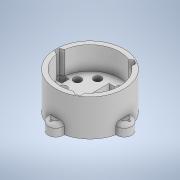
# Autodesk Inventor part: Enganche_H
Saved by Autodesk Inventor 2021 (Build 250183000, 183)
## iProperties
Created: 2021-10-28
Part Number: Enganche_H
Material: Genérico
Document SubType Name: Modeling
Designer: Joaquín
Density: 1 g/cm^3
Appearance: Valor por defecto
Author: Joaquín
Autodesk Inventor part; units mm, degrees
ref_plane "YZ Plane" through (0, 0, 0) normal (1, 0, 0) x (0, 1, 0)
ref_plane "XZ Plane" through (0, 0, 0) normal (0, 1, 0) x (-1, 0, 0)
ref_plane "XY Plane" through (0, 0, 0) normal (0, 0, 1) x (1, 0, 0)
sketch "Boceto3" plane through (0, 0, 0) normal (0, 1, 0) x (-1, 0, 0)
  line L0 (-22.9127, 29.686) -> (-23.0801, 29.976)
  line L1 (-23.0801, 29.976) -> (-22.6604, 29.249)
  line L2 (-19.0849, 38.0561) -> (-23.4151, 35.5561)
  line L3 (-23.0801, 29.976) -> (-23.4151, 35.5561)
  line L4 (-23.4151, 35.5561) -> (-19.0849, 38.0561)
  line L5 (-19.0849, 38.0561) -> (-14.4199, 34.976)
  line L6 (-14.4199, 34.976) -> (-14.0002, 34.249)
  line L7 (-22.6604, -29.249) -> (-23.0801, -29.976)
  line L8 (-22.6604, -29.249) -> (-23.0801, -29.976)
  line L9 (-23.0801, -29.976) -> (-23.4151, -35.5561)
  line L10 (-23.0801, -29.976) -> (-23.4151, -35.5561)
  line L11 (-23.4151, -35.5561) -> (-19.0849, -38.0561)
  line L12 (-23.4151, -35.5561) -> (-19.0849, -38.0561)
  line L13 (-19.0849, -38.0561) -> (-14.4199, -34.976)
  line L14 (-14.4199, -34.976) -> (-14.0002, -34.249)
  line L15 (-14.4199, -34.976) -> (-14.0002, -34.249)
  line L16 (36.6606, -5) -> (37.5, -5)
  line L17 (36.6606, -5) -> (37.5, -5)
  line L18 (37.5, -5) -> (42.5, -2.5)
  line L19 (37.5, -5) -> (42.5, -2.5)
  line L20 (42.5, 2.5) -> (37.5, 5)
  line L21 (42.5, -2.5) -> (42.5, 2.5)
  line L22 (42.5, 2.5) -> (37.5, 5)
  line L23 (37.5, 5) -> (36.6606, 5)
  line L24 (37.5, 5) -> (36.6606, 5)
  arc A0 (36.6606, 5) -> (-14.0002, 34.249) centre (0, 0) ccw
  arc A1 (-22.6604, 29.249) -> (-22.6604, -29.249) centre (0, 0) ccw
  arc A2 (-14.0002, -34.249) -> (36.6606, -5) centre (0, 0) ccw
  circle A3 centre (0, 0) radius 45
  point P0 (5, 25)
  dimension "d7" = 90
  constraints: 50 end point, 8 collinear, 6 point on circle, 4 centre point, 2 perpendicular, 1 coincident, 1 horizontal, 1 parallel
  measures "d7" diameter of A3
extrude "Extrusión2" add sketch "Boceto3" along normal blind 30
sketch "Boceto4" plane through (0, 0, 0) normal (0, -1, 0) x (1, 0, 0)
  circle A0 centre (0, 0) radius 45
  line L0 (-42.5, -2.5) -> (-37.5, -5) projected
  line L1 (-36.6606, -5) -> (-37.5, -5)
  line L2 (-37.5, -5) -> (-42.5, -2.5)
  line L3 (-42.5, 2.5) -> (-42.5, -2.5) projected
  line L4 (-42.5, -2.5) -> (-42.5, 2.5)
  line L5 (-37.5, 5) -> (-42.5, 2.5) projected
  line L6 (-42.5, 2.5) -> (-37.5, 5)
  line L7 (-37.5, 5) -> (-36.6606, 5)
  line L8 (14.4199, 34.976) -> (14.0002, 34.249) projected
  line L9 (14.0002, 34.249) -> (14.4199, 34.976)
  line L10 (19.0849, 38.0561) -> (14.4199, 34.976) projected
  line L11 (14.4199, 34.976) -> (19.0849, 38.0561)
  line L12 (23.4151, 35.5561) -> (19.0849, 38.0561) projected
  line L13 (19.0849, 38.0561) -> (23.4151, 35.5561)
  line L14 (23.0801, 29.976) -> (23.4151, 35.5561) projected
  line L15 (23.4151, 35.5561) -> (23.0801, 29.976)
  line L16 (22.6604, 29.249) -> (23.0801, 29.976) projected
  line L17 (23.0801, 29.976) -> (22.6604, 29.249)
  line L18 (14.0002, -34.249) -> (14.4199, -34.976)
  line L19 (19.0849, -38.0561) -> (23.4151, -35.5561) projected
  line L20 (14.4199, -34.976) -> (19.0849, -38.0561)
  line L21 (19.0849, -38.0561) -> (23.4151, -35.5561)
  line L22 (23.4151, -35.5561) -> (23.0801, -29.976) projected
  line L23 (23.4151, -35.5561) -> (23.0801, -29.976)
  line L24 (23.0801, -29.976) -> (22.6604, -29.249)
  arc A1 (-36.6606, 5) -> (-36.6606, -5) centre (0, 0) ccw
  arc A2 (14.0002, -34.249) -> (22.6604, -29.249) centre (0, 0) ccw
  arc A3 (22.6604, 29.249) -> (14.0002, 34.249) centre (0, 0) ccw
  constraints: 30 end point, 12 equal length, 6 point on circle, 4 centre point, 2 coincident, 1 horizontal
extrude "Extrusión3" add sketch "Boceto4" along normal blind 10
sketch "Boceto5" plane through (0, -10, 0) normal (0, -1, 0) x (1, 0, 0)
  line L0 (0, 0) -> (0, 20)
  line L1 (0, 20) -> (20, 20)
  line L2 (20, 20) -> (20, -20)
  line L3 (20, -20) -> (0, -20)
  line L4 (0, -20) -> (0, 0)
  dimension "d12" = 20
  dimension "d13" = 20
  dimension "d14" = 40
  dimension "d15" = 20
  constraints: 10 end point, 2 perpendicular, 1 point on line, 1 vertical
  measures "d12" distance of L0.start L0.end
  measures "d13" distance of L0.end L1.end
  measures "d14" distance of L1.end L2.end
  measures "d15" distance of L2.end L3.end
extrude "Extrusión4" cut sketch "Boceto5" against normal blind 10
sketch "Boceto6" plane through (0, -10, 0) normal (0, -1, 0) x (1, 0, 0)
  line L0 (-36.6606, -5) -> (-32.1, -5)
  line L1 (-32.1, -5) -> (-32.1, 5)
  line L2 (-32.1, 5) -> (-36.6606, 5)
  arc A0 (-36.6606, 5) -> (-36.6606, -5) centre (0, 0) ccw
  line L3 (22.6604, -29.249) -> (20.3801, -25.2994)
  arc A1 (14.0002, -34.249) -> (22.6604, -29.249) centre (0, 0) ccw
  line L4 (20.3801, -25.2994) -> (11.7199, -30.2994)
  line L5 (11.7199, -30.2994) -> (14.0002, -34.249)
  line L6 (14.0002, 34.249) -> (11.7199, 30.2994)
  arc A2 (22.6604, 29.249) -> (14.0002, 34.249) centre (0, 0) ccw
  line L7 (11.7199, 30.2994) -> (20.3801, 25.2994)
  line L8 (20.3801, 25.2994) -> (22.6604, 29.249)
  dimension "d19" = 10
  dimension "d22" = 360
  constraints: 18 end point, 6 point on circle, 3 centre point, 2 perpendicular, 1 coincident, 28 other
  measures "d19" distance of L0.end L1.end
extrude "Extrusión5" cut sketch "Boceto6" against normal blind 10
sketch "Boceto7" plane through (0, -10, 0) normal (0, -1, 0) x (1, 0, 0)
  circle A0 centre (27.5, 0) radius 2.5
  circle A1 centre (21.0662, 17.6767) radius 2.5
  circle A2 centre (4.7753, 27.0822) radius 2.5
  circle A3 centre (-13.75, 23.8157) radius 2.5
  circle A4 centre (-25.8415, 9.4056) radius 2.5
  circle A5 centre (-25.8415, -9.4056) radius 2.5
  circle A6 centre (-13.75, -23.8157) radius 2.5
  circle A7 centre (4.7753, -27.0822) radius 2.5
  circle A8 centre (21.0662, -17.6767) radius 2.5
  circle A9 centre (-13.75, -23.8157) radius 5
  circle A10 centre (-25.8415, -9.4056) radius 5
  circle A11 centre (-25.8415, 9.4056) radius 5
  circle A12 centre (-13.75, 23.8157) radius 5
  point P0 (0, 0)
  dimension "d29" = 5
  dimension "d32" = 360
  dimension "d34" = 10
  dimension "d35" = 10
  constraints: 13 centre point, 4 coincident, 19 other
  measures "d29" diameter of A0
  measures "d34" diameter of A9
  measures "d35" diameter of A10
extrude "Extrusión6" cut sketch "Boceto7" against normal blind 10 contours A3 | A4 | A5 | A6 | A9 | A10 | A11 | A12
sketch "Boceto10" plane through (0, 0, 0) normal (0, 1, 0) x (1, 0, 0)
  line L0 (0, 20) -> (0, -20) projected
  arc A0 (14.8215, -21.6306) -> (5.3674, -21.5551) centre (10.1075, -19.9639) ccw
  arc A1 (7.6437, -28.3362) -> (12.4372, -28.3744) centre (10.0471, -27.5294) ccw
  line L1 (12.4658, -28.2937) -> (14.8215, -21.6306)
  line L2 (7.6356, -28.3119) -> (5.3674, -21.5551)
  line L3 (12.4372, -28.3744) -> (12.4658, -28.2937)
  line L4 (7.6437, -28.3362) -> (7.6356, -28.3119)
  line L5 (20, -20) -> (0, -20) projected
  line L6 (20, 20) -> (0, 20) projected
  arc A2 (5.1785, 21.6306) -> (14.6326, 21.5551) centre (9.8925, 19.9639) ccw
  arc A3 (12.3563, 28.3362) -> (7.5628, 28.3744) centre (9.9529, 27.5294) ccw
  line L7 (7.5342, 28.2937) -> (5.1785, 21.6306)
  line L8 (12.3644, 28.3119) -> (14.6326, 21.5551)
  line L9 (7.5628, 28.3744) -> (7.5342, 28.2937)
  line L10 (12.3563, 28.3362) -> (12.3644, 28.3119)
  point P0 (0, 0)
  point P1 (10, 0)
  point P2 (7.5628, 28.3744)
  dimension "d49" = 10
  dimension "d53" = 360
  constraints: 16 end point, 8 point on circle, 4 centre point, 4 point on line, 4 tangent, 31 other
  measures "d49" diameter of A0
extrude "Extrusión7" cut sketch "Boceto10" against normal blind 12
sketch "Boceto13" plane through (0, -10, 0) normal (0, -1, 0) x (1, 0, 0)
  arc A0 (31, 10) -> (10.1128, 30.9997) centre (10, 10) ccw
  arc A1 (10.1128, -30.9997) -> (31, -10) centre (10, -10) ccw
  arc A2 (-8.4662, 0) -> (-11, -10) centre (10, -10) ccw
  line L0 (0, -20) -> (0, 20) projected
  line L1 (0, 10) -> (0, -10)
  arc A3 (-11, 10) -> (-8.4662, 0) centre (10, 10) ccw
  arc A4 (-9.2351, 12.3895) -> (-11, 10) centre (-8.5, 10) ccw
  line L2 (-1.5423, 14.7562) -> (-9.2351, 12.3895)
  line L3 (0, 15) -> (0, 8.4662)
  arc A5 (0, 15) -> (-1.5423, 14.7562) centre (0, 10) ccw
  arc A6 (-11, -10) -> (-8.5, -12.5) centre (-8.5, -10) ccw
  line L4 (-1.5423, -14.7562) -> (-9.2351, -12.3895)
  line L5 (0, -10) -> (0, -15)
  arc A7 (-1.5423, -14.7562) -> (0, -15) centre (0, -10) ccw
  arc A8 (20, 5) -> (21.5423, 5.2438) centre (20, 10) ccw
  arc A9 (21.5423, -5.2438) -> (20, -5) centre (20, -10) ccw
  arc A10 (31, -10) -> (28.5, -7.5) centre (28.5, -10) ccw
  arc A11 (28.5, 7.5) -> (31, 10) centre (28.5, 10) ccw
  line L6 (21.5423, -5.2438) -> (29.2351, -7.6105)
  line L7 (20, 20) -> (15.1073, 20) projected
  line L8 (21.5423, 5.2438) -> (29.2351, 7.6105)
  line L9 (20, 5) -> (20, -5)
  line L10 (20, 20) -> (20, -20) projected
  circle A12 centre (0, 0) radius 45
  circle A13 centre (-13.75, 23.8157) radius 5 projected
  circle A14 centre (-13.75, 23.8157) radius 5
  circle A15 centre (-25.8415, 9.4056) radius 5 projected
  circle A16 centre (-25.8415, 9.4056) radius 5
  circle A17 centre (-25.8415, -9.4056) radius 5 projected
  circle A18 centre (-25.8415, -9.4056) radius 5
  circle A19 centre (-13.75, -23.8157) radius 5 projected
  circle A20 centre (-13.75, -23.8157) radius 5
  arc A21 (7.5628, -28.3744) -> (12.3563, -28.3362) centre (9.9529, -27.5294) ccw projected
  line L11 (0, 15) -> (0, 20)
  line L12 (0, 20) -> (5.1076, 20) projected
  line L13 (0, 20) -> (5.1076, 20)
  arc A22 (15.1073, 20) -> (14.8215, 21.6306) centre (10.1075, 19.9639) ccw projected
  arc A23 (16.1074, 20) -> (16.1034, 20.1849) centre (10.1075, 19.9639) ccw
  arc A24 (10.1128, 30.9997) -> (7.2499, 29.5844) centre (10.0471, 27.5294) ccw
  line L14 (6.5761, 27.5294) -> (4.1076, 20)
  line L15 (4.1076, 20) -> (7.2499, 29.5844)
  arc A25 (7.2499, -29.5844) -> (10.1128, -30.9997) centre (10.0471, -27.5294) ccw
  line L16 (4.1076, -20) -> (7.2499, -29.5844)
  line L17 (0, 15) -> (0, 20)
  line L18 (4.1076, 20) -> (0, 20)
  line L19 (0, -15) -> (0, -20)
  line L20 (0, -20) -> (4.1076, -20)
  line L21 (0, -20) -> (4.8927, -20) projected
  constraints: 34 end point, 30 point on circle, 20 centre point, 8 coincident, 8 point on line, 7 collinear, 4 tangent, 1 midpoint, 1 vertical
extrude "Extrusión8" add sketch "Boceto13" along normal blind 8
sketch "Boceto14" plane through (0, -18, 0) normal (0, -1, 0) x (1, 0, 0)
  circle A0 centre (0, 0) radius 45
  circle A1 centre (-13.75, -23.8157) radius 5 projected
  circle A2 centre (-13.75, -23.8157) radius 5
  circle A3 centre (-25.8415, -9.4056) radius 5 projected
  circle A4 centre (-25.8415, -9.4056) radius 5
  circle A5 centre (-25.8415, 9.4056) radius 5 projected
  circle A6 centre (-25.8415, 9.4056) radius 5
  circle A7 centre (-13.75, 23.8157) radius 5 projected
  circle A8 centre (-13.75, 23.8157) radius 5
  constraints: 5 centre point, 5 coincident
extrude "Extrusión9" add sketch "Boceto14" along normal blind 8
sketch "Boceto15" plane through (0, -26, 0) normal (0, -1, 0) x (1, 0, 0)
  line L0 (0, -35) -> (20, -35)
  line L1 (0, 35) -> (20, 35)
  line L2 (35, 0) -> (35, -10)
  line L3 (35, 0) -> (35, 10)
  line L4 (0, -35) -> (0, -30)
  line L5 (20, -35) -> (20, -30)
  line L6 (20, -30) -> (0, -30)
  line L7 (35, -10) -> (30, -10)
  line L8 (30, -10) -> (30, 10)
  line L9 (30, 10) -> (35, 10)
  line L10 (20, 35) -> (20, 30)
  line L11 (20, 30) -> (0, 30)
  line L12 (0, 30) -> (0, 35)
  dimension "d86" = 20
  dimension "d87" = 20
  dimension "d91" = 5
  dimension "d92" = 5
  dimension "d93" = 5
  dimension "d94" = 5
  constraints: 26 end point, 5 vertical, 4 perpendicular, 3 horizontal
  measures "d86" distance of L0.start L0.end
  measures "d87" distance of L1.start L1.end
  measures "d91" distance of L0.start L4.end
  measures "d92" distance of L0.end L5.end
  measures "d93" distance of L2.end L7.end
  measures "d94" distance of L1.end L10.end
extrude "Extrusión10" add sketch "Boceto15" along normal blind 20
sketch "Boceto17" plane through (0, -26, 35) normal (0, 0, 1) x (1, 0, 0)
  circle A0 centre (5, -15) radius 1.5
  circle A1 centre (15, -15) radius 1.5
  circle A2 centre (10, -5) radius 1.5
  point P0 (0, 26)
  point P1 (0, -20)
  dimension "d118" = 3
  constraints: 3 centre point
  measures "d118" diameter of A2
extrude "Extrusión11" cut sketch "Boceto17" against normal blind 100
sketch "Boceto19" plane through (35, -26, 10) normal (1, 0, 0) x (0, 0, -1)
  circle A0 centre (5, -15) radius 1.5
  circle A1 centre (15, -15) radius 1.5
  circle A2 centre (10, -5) radius 1.5
  point P0 (10, 26)
  point P1 (0, -20)
  dimension "d114" = 3
  dimension "d115" = 3
  dimension "d116" = 3
  constraints: 3 centre point
  measures "d114" diameter of A0
  measures "d115" diameter of A1
  measures "d116" diameter of A2
extrude "Extrusión12" cut sketch "Boceto19" against normal blind 100
fillet "Empalme1" radius 2 3 edges at (-18.5, 30, 32.0429) (37, 30, 0) (-18.5, 30, -32.0429)
sketch "Boceto22" plane through (0, -46, 0) normal (0, -1, 0) x (1, 0, 0)
  circle A0 centre (80.4507, 56.8705) radius 177.5507
  point P0 (0, 0)
  constraints: 1 centre point
extrude "Extrusión13" cut sketch "Boceto22" against normal blind 28
sketch "Boceto23" plane through (0, -18, 0) normal (0, -1, 0) x (1, 0, 0)
  circle A0 centre (0, 0) radius 45 projected
  arc A1 (-9.9381, -43.8889) -> (9.9381, -43.8889) centre (0, -45) ccw
  circle A2 centre (0, -51) radius 1.5
  arc A3 (43.8889, -9.9381) -> (43.8889, 9.9381) centre (45, 0) ccw
  circle A4 centre (51, 0) radius 1.5
  arc A5 (9.9381, 43.8889) -> (-9.9381, 43.8889) centre (0, 45) ccw
  circle A6 centre (0, 51) radius 1.5
  arc A7 (-43.8889, 9.9381) -> (-43.8889, -9.9381) centre (-45, 0) ccw
  circle A8 centre (-51, 0) radius 1.5
  dimension "d133" = 360
  constraints: 11 point on circle, 8 centre point, 25 other
extrude "Extrusión14" add sketch "Boceto23" against normal blind 15 contours A0 A3 | A0 A5 | A1 A0 | A0 A7
fillet "Empalme2" radius 5 4 edges at (0, -3, -55) (55, -3, 0) (0, -3, 55) (-55, -3, 0)
sketch "Boceto24" plane through (0, 30, 0) normal (0, 1, 0) x (1, 0, 0)
  line L0 (-43.5, -2.5) -> (-43.5, 2.5)
  line L1 (-42.5, 3.5) -> (-37.5, 6)
  line L2 (-42.5, -3.5) -> (-37.5, -6)
  line L3 (-37.5, -6) -> (-32.1, -6)
  line L4 (-31.1, -5) -> (-31.1, -6)
  line L5 (-31.1, -6) -> (-32.1, -6)
  line L6 (-31.1, -5) -> (-31.1, 5)
  line L7 (-32.1, 6) -> (-31.1, 6)
  line L8 (-31.1, 6) -> (-31.1, 5)
  line L9 (-32.1, 6) -> (-37.5, 6)
  line L10 (-43.5, 2.5) -> (-43.5, 3)
  line L11 (-42.5, 3.5) -> (-43.5, 3)
  line L12 (-42.5, -3.5) -> (-43.5, -3)
  line L13 (-43.5, -3) -> (-43.5, -2.5)
  line L14 (18.2189, -38.5561) -> (19.1519, -39.1721)
  line L15 (19.5849, -38.9221) -> (19.1519, -39.1721)
  line L16 (23.9151, -36.4221) -> (19.5849, -38.9221)
  line L17 (24.3481, -36.1721) -> (23.9151, -36.4221)
  line L18 (24.2811, -35.0561) -> (24.3481, -36.1721)
  line L19 (18.2189, -38.5561) -> (13.5538, -35.476)
  line L20 (24.2811, -35.0561) -> (23.9462, -29.476)
  line L21 (10.8538, -30.7994) -> (13.5538, -35.476)
  line L22 (10.8538, -30.7994) -> (10.3538, -29.9334)
  line L23 (10.3538, -29.9334) -> (11.2199, -29.4334)
  line L24 (19.8801, -24.4334) -> (11.2199, -29.4334)
  line L25 (23.9462, -29.476) -> (21.2462, -24.7994)
  line L26 (19.8801, -24.4334) -> (20.7462, -23.9334)
  line L27 (20.7462, -23.9334) -> (21.2462, -24.7994)
  line L28 (24.2811, 35.0561) -> (24.3481, 36.1721)
  line L29 (23.9151, 36.4221) -> (24.3481, 36.1721)
  line L30 (19.5849, 38.9221) -> (23.9151, 36.4221)
  line L31 (19.1519, 39.1721) -> (19.5849, 38.9221)
  line L32 (18.2189, 38.5561) -> (19.1519, 39.1721)
  line L33 (24.2811, 35.0561) -> (23.9462, 29.476)
  line L34 (18.2189, 38.5561) -> (13.5538, 35.476)
  line L35 (21.2462, 24.7994) -> (23.9462, 29.476)
  line L36 (21.2462, 24.7994) -> (20.7462, 23.9334)
  line L37 (20.7462, 23.9334) -> (19.8801, 24.4334)
  line L38 (11.2199, 29.4334) -> (19.8801, 24.4334)
  line L39 (13.5538, 35.476) -> (10.8538, 30.7994)
  line L40 (11.2199, 29.4334) -> (10.3538, 29.9334)
  line L41 (10.3538, 29.9334) -> (10.8538, 30.7994)
  circle A0 centre (0, 0) radius 39
  point P0 (-42.5, -2.5)
  point P1 (-42.5, 2.5)
  point P2 (-37.5, 5)
  point P3 (-32.1, -5)
  point P4 (-32.1, 5)
  point P5 (-37.5, -5)
  point P6 (23.4151, -35.5561)
  point P7 (19.0849, -38.0561)
  point P8 (14.4199, -34.976)
  point P9 (23.0801, -29.976)
  point P10 (11.7199, -30.2994)
  point P11 (20.3801, -25.2994)
  point P12 (19.0849, 38.0561)
  point P13 (23.4151, 35.5561)
  point P14 (23.0801, 29.976)
  point P15 (14.4199, 34.976)
  point P16 (20.3801, 25.2994)
  point P17 (11.7199, 30.2994)
  point P18 (24.0211, -30.7244)
  point P19 (14.5975, -36.1651)
  point P20 (14.5975, 36.1651)
  point P21 (24.0211, 30.7244)
  point P22 (-38.6186, -5.4407)
  point P23 (-38.6186, 5.4407)
  dimension "d149" = 360
  constraints: 84 end point, 3 perpendicular, 3 point on line, 3 vertical, 1 centre point, 1 coincident, 1 horizontal, 103 other
extrude "Extrusión15" cut sketch "Boceto24" against normal blind 30 contours L0 L10 L11 L1 A0 L2 L12 L13 | L2 L3 L5 L4 L6 L8 L7 L9 L1 A0 L34 L39 L41 L40 L38 L37 L36 L35 L33 L20 L25 L27 L26 L24 L23 L22 L21 L19 | A0 L20 L18 L17 L16 L15 L14 L19 | L34 L32 L31 L30 L29 L28 L33 A0
sketch "Boceto25" plane through (0, 30, 0) normal (0, 1, 0) x (1, 0, 0)
  circle A0 centre (0, 0) radius 39
  constraints: 1 centre point, 1 coincident
extrude "Extrusión16" cut sketch "Boceto25" against normal blind 30
sketch "Boceto27" plane through (0, 0, 0) normal (0, 1, 0) x (1, 0, 0)
  line L0 (20, -21) -> (0, -21)
  line L1 (-1, -20) -> (-1, 20)
  line L2 (0, 21) -> (20, 21)
  line L3 (21, 20) -> (21, -20)
  line L4 (21, -21) -> (21, -20)
  line L5 (21, -21) -> (20, -21)
  line L6 (0, -21) -> (-1, -21)
  line L7 (-1, -21) -> (-1, -20)
  line L8 (-1, 20) -> (-1, 21)
  line L9 (-1, 21) -> (0, 21)
  line L10 (20, 21) -> (21, 21)
  line L11 (21, 21) -> (21, 20)
  point P0 (0, 0)
  point P1 (0, -20)
  point P2 (0, 20)
  point P3 (20, -20)
  constraints: 24 end point, 3 horizontal, 3 perpendicular, 3 vertical, 2 point on line, 1 collinear
extrude "Extrusión17" cut sketch "Boceto27" against normal blind 20
sketch "Boceto28" plane through (0, 0, 0) normal (0, 1, 0) x (1, 0, 0)
  line L0 (21, 21) -> (21, -21) projected
  line L1 (21, 21) -> (21, 26)
  line L2 (21, 26) -> (-1, 26)
  line L3 (-1, -21) -> (-1, 21) projected
  line L4 (-1, 26) -> (-1, 21)
  line L5 (-1, -21) -> (-1, -26)
  line L6 (21, -21) -> (21, -26)
  line L7 (21, -26) -> (-1, -26)
  line L8 (-1, -21) -> (4.4354, -21) projected
  line L9 (21, -21) -> (-1, -21)
  line L10 (21, 21) -> (-1, 21)
  point P0 (0, 0)
  dimension "d171" = 5
  dimension "d172" = 5
  dimension "d173" = 5
  constraints: 16 end point, 3 vertical, 2 horizontal, 2 perpendicular
  measures "d171" distance of L0.start L1.end
  measures "d172" distance of L3.start L5.end
  measures "d173" distance of L0.end L6.end
extrude "Extrusión18" cut sketch "Boceto28" against normal blind 20 contours L10 L4 L2 L1 | L6 L7 L5 L8 L9
sketch "Boceto30" plane through (0, -10, 0) normal (0, -1, 0) x (1, 0, 0)
  arc A0 (12.4372, 28.3744) -> (7.6437, 28.3362) centre (10.0471, 27.5294) ccw projected
  arc A1 (12.0656, 30.8982) -> (10.1128, 30.9997) centre (10, 10) ccw projected
  arc A2 (10.1128, 30.9997) -> (7.2499, 29.5844) centre (10.0471, 27.5294) ccw
  arc A3 (10.1128, 30.9997) -> (7.2499, 29.5844) centre (10.0471, 27.5294) ccw projected
  line L0 (7.2499, 29.5844) -> (6.0747, 26) projected
  line L1 (7.2499, 29.5844) -> (6.0747, 26)
  line L2 (6.0747, 26) -> (6.8595, 26)
  line L3 (6.8595, 26) -> (6.0747, 26)
  arc A4 (12.0656, 30.8982) -> (10, 31) centre (10, 10) ccw
  line L4 (11.7199, 30.2994) -> (12.0656, 30.8982) projected
  line L5 (12.0656, 30.8982) -> (11.7199, 30.2994)
  line L6 (11.7199, 30.2994) -> (19.1667, 26)
  line L7 (19.1667, 26) -> (13.2767, 26) projected
  line L8 (19.1667, 26) -> (13.2767, 26)
  line L9 (13.2767, 26) -> (12.4372, 28.3744)
  line L10 (7.6437, 28.3362) -> (6.8595, 26)
  arc A5 (12.4372, 28.3744) -> (7.6437, 28.3362) centre (10.0471, 27.5294) ccw
  arc A6 (10.1128, -30.9997) -> (12.0656, -30.8982) centre (10, -10) ccw
  arc A7 (7.2499, -29.5844) -> (10.1128, -30.9997) centre (10.0471, -27.5294) ccw
  arc A8 (7.2499, -29.5844) -> (10.1128, -30.9997) centre (10.0471, -27.5294) ccw
  line L11 (7.2499, -29.5844) -> (6.0747, -26)
  line L12 (7.2499, -29.5844) -> (6.0747, -26)
  arc A9 (10, -31) -> (12.0656, -30.8982) centre (10, -10) ccw
  line L13 (11.7199, -30.2994) -> (12.0656, -30.8982)
  line L14 (12.0656, -30.8982) -> (11.7199, -30.2994)
  line L15 (11.7199, -30.2994) -> (19.1667, -26)
  line L16 (19.1667, -26) -> (13.2767, -26)
  line L17 (19.1667, -26) -> (13.2767, -26)
  line L18 (-1, -26) -> (6.7233, -26) projected
  line L19 (6.0747, -26) -> (6.7233, -26)
  line L20 (19.1667, -26) -> (13.1405, -26) projected
  line L21 (13.2767, -26) -> (13.1405, -26)
  arc A10 (7.8572, -28.8067) -> (12.578, -27.6757) centre (10.0471, -27.5294) ccw
  line L22 (13.1405, -26) -> (12.578, -27.6757)
  line L23 (13.1405, -26) -> (12.3563, -28.3362) projected
  line L24 (6.7233, -26) -> (7.5628, -28.3744) projected
  line L25 (6.7233, -26) -> (7.5628, -28.3744)
  line L26 (7.5628, -28.3744) -> (7.8572, -28.8067)
  point P0 (0, 0)
  point P1 (10.1128, 30.9997)
  point P2 (10, 31)
  constraints: 40 end point, 22 point on circle, 8 centre point, 6 collinear, 4 coincident, 1 concentric, 1 horizontal, 1 perpendicular, 1 point on line
extrude "Extrusión19" cut sketch "Boceto30" against normal blind 20
sketch "Boceto31" plane through (0, -10, 0) normal (0, -1, 0) x (1, 0, 0)
  circle A0 centre (11.8103, -26.5181) radius 4.1443
  point P0 (0, 0)
  constraints: 1 centre point
extrude "Extrusión20" cut sketch "Boceto31" against normal blind 20
